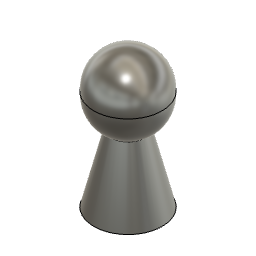
MMEZP_Figurka v1 (Autodesk Fusion 360 design; units mm, degrees)
Autodesk Fusion 360 part; units mm, degrees
sketch "Sketch3" plane through (0, 0, 0) normal (0, 1, 0) x (1, 0, 0)
  circle A0 centre (0, 0) radius 2.5
  dimension "d5" = 5
  constraint coincident A0.centre origin
  measures "d5" diameter of A0
extrude "Extrude2" add sketch "Sketch3" along normal blind 10 makes body 1
draft "Draft1" angle 14 neutral plane through (0, 10, 0) pull (0, 1, 0) 1 faces at (2.4969, 6.6667, 0.1246) on bodies 1
sketch "Sketch4" plane through (0, 10, 0) normal (0, 1, 0) x (-1, 0, 0)
  circle A0 centre (0, 0) radius 2.5
  circle A1 centre (0, 0) radius 5
  dimension "d10" = 10
  constraint concentric A0 A1
  measures "d10" diameter of A1
extrude "Extrude3" add sketch "Sketch4" along normal blind 10 separate body makes body 2
extrude "Extrude4" add 1 faces at (-0.7508, 10, -0.3616) along direction (0, 1, 0) blind 10 on bodies 1 bodies 1 2
fillet "Fillet1" radius 5 1 edges at (4.6616, 20, -1.8081) on bodies 1
fillet "Fillet2" radius 5 1 edges at (4.6616, 10, -1.8081) on bodies 1
delete_face "DeleteFace1" 1 faces at (-4.9752, 14.7767, -0.4978) on bodies 1
